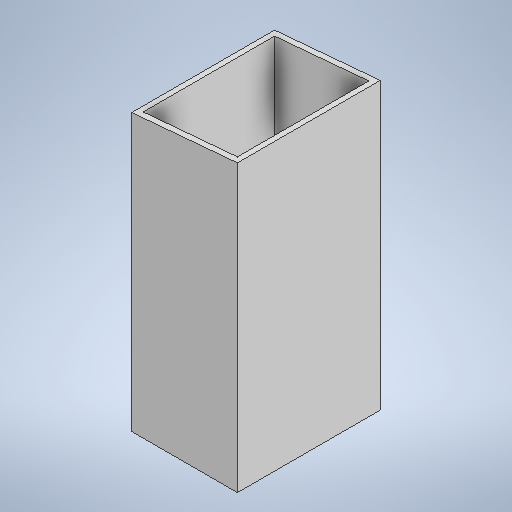
# Autodesk Inventor part: Housing of the motor
Saved by Autodesk Inventor 2025 (Build 290162000, 162)
## iProperties
Created: 2026-04-10
Part Number: Housing of the motor
Material: Generic
Document SubType Name: Modeling
Designer: lenovo
Density: 1 g/cm^3
Appearance: Default
Author: lenovo
Autodesk Inventor part; units mm, degrees
ref_plane "YZ Plane" through (0, 0, 0) normal (1, 0, 0) x (0, 1, 0)
ref_plane "XZ Plane" through (0, 0, 0) normal (0, 1, 0) x (-1, 0, 0)
ref_plane "XY Plane" through (0, 0, 0) normal (0, 0, 1) x (1, 0, 0)
sketch "Sketch1" plane through (0, 0, 0) normal (0, 0, 1) x (1, 0, 0)
  line L0 (0, 0) -> (37, 0)
  line L1 (37, 0) -> (37, 100)
  line L2 (0, 96.7629) -> (0, 0)
  line L3 (37, 100) -> (0, 96.7629)
  line L4 (37, 100) -> (74.1413, 100) construction
  dimension "d0" = 37
  dimension "d1" = 100
  dimension "d2" = 175
  constraints: 10 end point, 2 horizontal, 1 equal length, 1 perpendicular
  measures "d0" distance of L0.start L0.end
  measures "d1" distance of L0.end L1.end
  measures "d2" angle of L3 L4
extrude "Extrusion1" add sketch "Sketch1" along normal blind 50
sketch "Sketch2" plane through (0, 0, 0) normal (0, -1, 0) x (1, 0, 0)
  line L0 (35, 48) -> (35, 2)
  line L1 (37, 0) -> (0, 0) projected
  line L2 (35, 2) -> (2, 2)
  line L3 (2, 2) -> (2, 48)
  line L4 (2, 48) -> (35, 48)
  dimension "d5" = 46
  dimension "d6" = 33
  constraints: 8 end point, 3 perpendicular, 1 horizontal
  measures "d5" distance of L0.start L0.end
  measures "d6" distance of L0.end L2.end
extrude "Extrusion2" cut sketch "Sketch2" against normal blind 100
body "Solid1"
